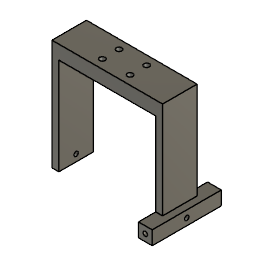
part - head2 (Autodesk Fusion 360 design; units mm, degrees)
Autodesk Fusion 360 part; units mm, degrees
note: some values were not read from the file. Set by a fixed rule: which sketch regions a step uses.
sketch "Sketch3" plane through (0, 0, 0) normal (0, 1, 0) x (1, 0, 0)
  line L0 (40, -40) -> (-40, -40)
  line L1 (-40, -40) -> (-40, 40)
  line L2 (-40, 40) -> (40, 40)
  line L3 (40, 40) -> (40, -40)
  line L4 (40, -40) -> (-40, 40) construction
  line L5 (-40, -40) -> (40, 40) construction
  line L6 (35, 49.9978) -> (35, -35)
  line L7 (35, -35) -> (-35, -35)
  line L8 (-35, -35) -> (-35, 49.9995)
  dimension "d45" = 80
  dimension "d46" = 80
  dimension "d47" = 5
  constraint horizontal L0
  constraint perpendicular L0 L1
  constraint parallel L0 L2
  constraint parallel L1 L3
  constraint coincident L4 origin
  constraint coincident L5 origin
  measures "d45" distance of L0.start L0.end
  measures "d46" distance of L0.end L1.end
extrude "Extrude10" add sketch "Sketch3" along normal mid plane 25 contours L0 L1 L2 L3 L6 L7 L8
sketch "Sketch9" plane through (40, 0, 0) normal (1, 0, 0) x (0, 1, 0)
  line L0 (-12.5, -40) -> (12.5, -40)
  line L1 (12.5, -40) -> (12.5, 40)
  line L2 (12.5, 40) -> (-12.5, 40)
  line L3 (-12.5, 40) -> (-12.5, -40)
  line L4 (25, -40) -> (-25, -40)
  line L5 (-25, -40) -> (-25, -30)
  line L6 (-25, -30) -> (25, -30)
  line L7 (25, -30) -> (25, -40)
  line L8 (25, -40) -> (-25, -30) construction
  line L9 (-25, -40) -> (25, -30) construction
  line L10 (0, -30.1567) -> (0, 30.1567)
  point P0 (0, -35)
  dimension "d50" = 10
  dimension "d51" = 5
  dimension "d52" = 25
  dimension "d53" = 50
  constraint horizontal L4
  constraint perpendicular L4 L5
  constraint parallel L4 L6
  constraint parallel L5 L7
  constraint coincident L8 P0
  constraint coincident L9 P0
  constraint midpoint L10 origin
  constraint parallel L3 L10
  measures "d50" distance of L4 L6
  measures "d51" distance of L0 P0
  measures "d52" distance of L5 L10
  measures "d53" distance of L5.end L6.end
extrude "Extrude11" add sketch "Sketch9" along normal mid plane 10 contours L0 L1 L3 L4 L6 | L3 L4 L5 L6 | L1 L4 L6 L7
sketch "Sketch10" plane through (0, -25, 0) normal (0, -1, 0) x (1, 0, 0)
  line L0 (35, -40) -> (45, -40)
  line L1 (45, -40) -> (45, -30)
  line L2 (45, -30) -> (35, -30)
  line L3 (35, -30) -> (35, -40)
  line L4 (35, -40) -> (45, -30)
  line L5 (45, -40) -> (40, -35)
  circle A0 centre (40, -35) radius 1.6
  dimension "d56" = 3.2
  constraint coincident L0.start L3.end
  constraint coincident L1.end L2.start
  constraint coincident L0.end L1.start
  constraint midpoint L4 L5.end
  constraint coincident L5.end A0.centre
  measures "d56" diameter of A0
extrude "Extrude12" cut sketch "Sketch10" against normal blind 64 contours L4 A0 | L4 L5 A0 | L4 L5 A0
sketch "Sketch11" plane through (45, 0, 0) normal (1, 0, 0) x (0, 1, 0)
  line L0 (25, -30) -> (-25, -30)
  line L1 (-25, -30) -> (-25, -40)
  line L2 (-25, -40) -> (25, -40)
  line L3 (25, -40) -> (25, -30)
  line L4 (-25, -40) -> (25, -30)
  line L5 (25, -40) -> (-25, -30)
  circle A0 centre (0, -35) radius 1.6
  dimension "d59" = 3.2
  constraint coincident L1.end L2.start
  constraint coincident L0.start L3.end
  constraint coincident L2.end L3.start
  constraint coincident L0.end L1.start
  constraint midpoint L4 A0.centre
  measures "d59" diameter of A0
extrude "Extrude13" cut sketch "Sketch11" against normal blind 105 contours L4 L5 A0 | L4 L5 A0 | L4 L5 A0 | L4 L5 A0
extrude "Extrude14" add 1 faces at (11.6667, -4.1667, 35) along direction (0, 0, -1) blind 5
sketch "Sketch12" plane through (0, 0, 40) normal (0, 0, 1) x (-1, 0, 0)
  line L0 (-40, 12.5) -> (-40, -12.5)
  line L1 (-40, -12.5) -> (40, -12.5)
  line L2 (40, -12.5) -> (40, 12.5)
  line L3 (40, 12.5) -> (-40, 12.5)
  circle A0 centre (10, -6) radius 2
  circle A1 centre (-10, -6) radius 2
  circle A2 centre (10, 6) radius 2
  circle A3 centre (-10, 6) radius 2
  dimension "d68" = 4
  dimension "d69" = 10
  dimension "d70" = 6
  dimension "d73" = -20
  dimension "d74" = 12
  measures "d68" diameter of A0
  measures "d69" horizontal distance of origin A0.centre
  measures "d70" vertical distance of origin A0.centre
extrude "Extrude15" cut sketch "Sketch12" against normal blind 5.5 contours A0 | A1 | A2 | A3
equation "d48 = ( 25 / 2 ) * 1 mm"
